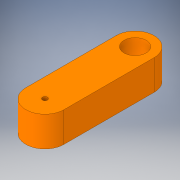
# Autodesk Inventor part: ArmThicker
Saved by Autodesk Inventor 2017 (Build 210142000, 142)
## iProperties
Created: 2017-03-25
Part Number: ArmThicker
Material: Generic
Document SubType Name: Modeling
Designer: Parshant Bombhi
Density: 1 g/cm^3
Appearance: Default
LengthOfArm_Thicker: 128.000 mm
Thickness_Thicker: 30.000 mm
Author: Parshant Bombhi
Autodesk Inventor part; units mm, degrees
ref_plane "YZ Plane" through (0, 0, 0) normal (1, 0, 0) x (0, 1, 0)
ref_plane "XZ Plane" through (0, 0, 0) normal (0, 1, 0) x (-1, 0, 0)
ref_plane "XY Plane" through (0, 0, 0) normal (0, 0, 1) x (1, 0, 0)
sketch "Sketch1" plane through (0, 0, 0) normal (0, 1, 0) x (-1, 0, 0)
  line L0 (0, -19) -> (0, -109)
  line L1 (19, -128) -> (19, -128)
  line L2 (38, -109) -> (38, -19)
  line L3 (19, 0) -> (19, 0)
  arc A0 (0, -109) -> (19, -128) centre (19, -109) ccw
  arc A1 (19, -128) -> (38, -109) centre (19, -109) ccw
  arc A2 (38, -19) -> (19, 0) centre (19, -19) ccw
  arc A3 (19, 0) -> (0, -19) centre (19, -19) ccw
  circle A4 centre (19, -19) radius 2.5
  circle A5 centre (19, -109) radius 11
  point P0 (0, 0)
  point P1 (0, -128)
  point P2 (38, -128)
  dimension "d0" = 38
  dimension "LengthOfArm_Thicker" = 128
  dimension "d2" = 19
  dimension "d3" = 5
  dimension "d4" = 22
  constraints: 8 end point, 8 point on circle, 8 tangent, 6 centre point, 6 point on line, 3 equal radius, 3 perpendicular, 2 coincident, 1 vertical
  measures "d0" distance of point (0, -128) point (38, -128)
  measures "LengthOfArm_Thicker" distance of point (0, 0) point (0, -128)
  measures "d2" radius of A0
  measures "d3" diameter of A4
  measures "d4" diameter of A5
extrude "Extrusion1" add sketch "Sketch1" along normal blind 30
body "Solid1"
